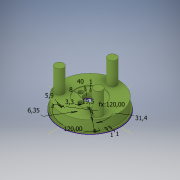
# Autodesk Inventor part: Output
Saved by Autodesk Inventor 2018.3 (Build 223284000, 284)
## iProperties
Created: 2018-07-20
Part Number: Output
Material: Generisch
Document SubType Name: Modeling
Designer: JochenAlt
Density: 1 g/cm^3
Appearance: Olivgrün
Author: JochenAlt
Autodesk Inventor part; units mm, degrees
ref_plane "YZ Plane" through (0, 0, 0) normal (1, 0, 0) x (0, 1, 0)
ref_plane "XZ Plane" through (0, 0, 0) normal (0, 1, 0) x (-1, 0, 0)
ref_plane "XY Plane" through (0, 0, 0) normal (0, 0, 1) x (1, 0, 0)
sketch "Skizze1" plane through (0, 0, 0) normal (0, 0, 1) x (1, 0, 0)
  line L0 (-29.4, 0) -> (29.4, 0) construction
  circle A0 centre (0, 0) radius 15.7 construction
  line L1 (0, 0) -> (-13.5966, -7.85) construction
  line L2 (0, 0) -> (13.5966, -7.85) construction
  line L3 (0, 29.4) -> (0, -29.4) construction
  line L4 (0, 0) -> (0, 15.7) construction
  circle A1 centre (0, 0) radius 9.75
  circle A2 centre (0, 0) radius 20
  circle A3 centre (0, 0) radius 6.35 construction
  circle A4 centre (-6.35, 0) radius 1.65
  circle A5 centre (0, 6.35) radius 1.65
  circle A6 centre (6.35, 0) radius 1.65
  circle A7 centre (0, -6.35) radius 1.65
  circle A8 centre (0, 0) radius 21
  circle A9 centre (0, 0) radius 21
  circle A10 centre (-13.5966, -7.85) radius 2.95
  circle A11 centre (0, 15.7) radius 2.95
  circle A12 centre (13.5966, -7.85) radius 2.95
  circle A13 centre (0, 0) radius 19
  circle A14 centre (0, 0) radius 4
  dimension "d1" = 31.4
  dimension "d2" = 120
  dimension "d13" = 120
  dimension "d14" = 19.5
  dimension "d16" = 40
  dimension "d21" = 6.35
  dimension "d22" = 3.3
  dimension "d26" = 1
  dimension "d27" = 1
  dimension "d30" = 5.9
  dimension "d33" = 1
  dimension "d42" = 8
  constraints: 15 centre point, 8 coincident, 6 end point, 6 point on circle, 6 point on line, 5 equal radius, 1 midpoint, 1 other
  measures "d1" diameter of A0
  measures "d2" angle of L2 L1
  measures "d13" angle of L4 L2
  measures "d14" diameter of A1
  measures "d16" diameter of A2
  measures "d21" radius of A3
  measures "d22" diameter of A4
  measures "d26" radial gap between concentric circles of A8 A2
  measures "d27" radial gap between concentric circles of A9 A2
  measures "d30" diameter of A10
  measures "d33" radial gap between concentric circles of A2 A13
  measures "d42" diameter of A14
extrude "Extrusion1" add sketch "Skizze1" along normal blind 1 contours A1 | A2 | A4 | A5 | A6 | A7 | A8 | A10 | A11 | A12 | A13 | A14
extrude "Extrusion3" add sketch "Skizze1" along normal blind 7 from surface at 1 contours A1 | A2 | A4 | A5 | A6 | A7 | A10 | A11 | A12 | A13 | A14
extrude "Extrusion8" add sketch "Skizze1" along normal blind 16 from surface at 8 contours A10 | A11 | A12
extrude "Extrusion9" cut sketch "Skizze1" along normal blind 5 contours A1 | A4 | A5 | A6 | A7 | A14
extrude "Extrusion10" cut sketch "Skizze1" along normal through all contours A4 | A5 | A6 | A7 | A14
extrude "Extrusion11" cut sketch "Skizze1" against normal blind 0.5 from surface at 8 contours A1 | A4 | A5 | A6 | A7 | A14
equation "\"d13\" = d2"
